Autodesk Fusion 360 part; units mm, degrees
note: some values were not read from the file. Set by a fixed rule: which sketch regions a step uses.
(part 3 of 3)
  constraint coincident P15 L924
  constraint tangent L923 A420
  constraint tangent L924 A420
  constraint tangent L926 A421
  constraint tangent L927 A421
  constraint equal A420 A421
  constraint coincident P17 L925
  constraint coincident P17 L926
  constraint tangent L925 A422
  constraint tangent L926 A422
  constraint equal A420 A422
  constraint coincident P16 L924
  constraint coincident P16 L925
  constraint tangent L924 A423
  constraint tangent L925 A423
  constraint equal A420 A423
  constraint tangent A79 L932
  constraint concentric A411 A424
  constraint tangent A413 A424
  constraint concentric A417 A427
  constraint concentric A418 A426
  constraint concentric A419 A425
  constraint concentric A412 A428
  constraint vertical L933
  constraint tangent A424 L934
  constraint vertical L934
  constraint perpendicular L929 L935
  constraint tangent L936 A426
  constraint coincident L938.start A428
  constraint tangent L938 A428
  constraint horizontal L938
  constraint concentric A428 A429
  constraint tangent L933 A430
  constraint tangent A427 A430
  constraint tangent L933 A431
  constraint tangent A426 A431
  constraint tangent L935 A432
  constraint tangent A425 A432
  constraint tangent L934 A433
  constraint tangent L935 A433
  constraint tangent L943 A441
  constraint perpendicular L926 L943
  constraint tangent L944 A441
  constraint perpendicular L926 L944
  constraint tangent L945 A443
  constraint tangent L946 A443
  constraint concentric A416 A448
  constraint tangent L937 A448
  constraint tangent A429 L951
  constraint vertical L951
  constraint perpendicular L951 L952
  constraint tangent L952 A449
  constraint tangent A448 A449
  constraint tangent L951 A450
  constraint tangent L952 A450
  constraint perpendicular L966 L967
  constraint perpendicular L963 L967
  constraint perpendicular L964 L966
  constraint tangent L966 A469
  constraint tangent A469 L967
  constraint tangent L964 A468
  constraint tangent A468 L965
  constraint equal A468 A469
  constraint tangent L963 A467
  constraint tangent A467 L964
  constraint equal A467 A469
  constraint tangent L967 A470
  constraint tangent L963 A470
  constraint equal A469 A470
  constraint tangent L974 A478
  constraint perpendicular L964 L974
  constraint tangent A478 L975
  constraint perpendicular L964 L975
  constraint tangent L972 A476
  constraint tangent A476 L973
  constraint horizontal L977
  constraint vertical L978
  constraint horizontal L979
  constraint vertical L976
  constraint concentric A483 A492
  constraint concentric A480 A491
  constraint concentric A489 A494
  constraint concentric A486 A493
  constraint tangent L976 A482
  constraint tangent A482 A483
  constraint tangent A483 A484
  constraint tangent A484 L977
  constraint equal A482 A484
  constraint tangent A481 L976
  constraint tangent A480 A481
  constraint equal A481 A482
  constraint tangent A479 L979
  constraint tangent A479 A480
  constraint equal A479 A482
  constraint tangent A490 L979
  constraint tangent A489 A490
  constraint equal A482 A490
  constraint tangent L978 A488
  constraint tangent A488 A489
  constraint equal A482 A488
  constraint tangent A486 A487
  constraint tangent A487 L978
  constraint equal A482 A487
  constraint tangent A485 A486
  constraint tangent L977 A485
  constraint equal A482 A485
  constraint horizontal L984
  constraint vertical L985
  constraint horizontal L986
  constraint vertical L987
  constraint tangent L987 A511
  constraint tangent L984 A511
  constraint tangent L986 A512
  constraint tangent L987 A512
  constraint equal A511 A512
  constraint tangent L985 A513
  constraint tangent L986 A513
  constraint equal A511 A513
  constraint tangent L984 A514
  constraint tangent L985 A514
  constraint equal A511 A514
  measures "d35" radius of A2
  measures "d36" radius of A3
  measures "d40" distance of L16.start L16.end
  measures "d41" radius of A4
  measures "d67" radius of A23
  measures "d68" distance of L75.start L75.end
  measures "d69" radius of A27
  measures "d89" radius of A39
  measures "d94" radius of A40
  measures "d112" diameter of A42
  measures "d113" diameter of A43
  measures "d116" radius of A46
  measures "d369" radius of A64
  measures "d426" diameter of A86
  measures "d427" diameter of A87
  measures "d429" radius of A88
  measures "d466" radius of A92
  measures "d474" radius of A94
  measures "d508" radius of A96
  measures "d524" diameter of A103
  measures "d525" diameter of A102
  measures "d526" radius of A104
  measures "d527" radius of A106
  measures "d528" radius of A108
  measures "d529" radius of A110
  measures "d532" distance of L341.start L341.end
  measures "d533" distance of L341.start L343.end
  measures "d534" distance of L345.start L345.end
  measures "d535" distance of L345.start L347.end
  measures "d545" radius of A116
  measures "d546" radius of A118
  measures "d555" radius of A130
  measures "d557" radius of A139
  measures "d579" radius of A171
  measures "d589" distance of L564.start L564.end
  measures "d591" radius of A172
  measures "d592" radius of A173
  measures "d593" radius of A174
  measures "d594" radius of A175
  measures "d604" radius of A182
  measures "d605" radius of A183
  measures "d643" radius of A186
  measures "d648" radius of A194
  measures "d652" radius of A205
  measures "d654" radius of A224
  measures "d655" radius of A225
  measures "d675" radius of A228
  measures "d686" radius of A230
  measures "d687" radius of A232
  measures "d688" distance of L676.start L713.end
  measures "d693" diameter of A273
  measures "d694" diameter of A274
  measures "d695" diameter of A275
  measures "d701" diameter of A276
  measures "d703" diameter of A278
  measures "d704" diameter of A279
  measures "d705" diameter of A280
  measures "d706" diameter of A281
  measures "d707" diameter of A282
  measures "d709" radius of A283
  measures "d718" diameter of A298
  measures "d719" diameter of A299
  measures "d722" radius of A300
  measures "d726" diameter of A308
  measures "d727" diameter of A309
  measures "d728" diameter of A310
  measures "d729" radius of A311
  measures "d742" radius of A348
  measures "d772" diameter of A369
  measures "d773" radius of A371
  measures "d774" radius of A381
  measures "d861" diameter of A394
  measures "d862" diameter of A395
  measures "d863" diameter of A396
  measures "d864" diameter of A397
  measures "d865" radius of A402
  measures "d872" diameter of A410
  measures "d873" diameter of A411
  measures "d876" diameter of A412
  measures "d882" radius of A413
  measures "d899" distance of L923.start P15
  measures "d901" distance of P16 P17
  measures "d902" radius of A420
  measures "d910" diameter of A427
  measures "d912" diameter of A426
  measures "d913" diameter of A425
  measures "d914" diameter of A428
  measures "d916" radius of A432
  measures "d918" radius of A433
  measures "d921" diameter of A440
  measures "d922" diameter of A441
  measures "d923" diameter of A442
  measures "d924" diameter of A443
  measures "d925" radius of A449
  measures "d926" radius of A450
  measures "d927" radius of A469
  measures "d928" diameter of A477
  measures "d929" diameter of A478
  measures "d930" diameter of A475
  measures "d931" diameter of A476
  measures "d932" diameter of A492
  measures "d933" diameter of A493
  measures "d934" diameter of A491
  measures "d935" diameter of A494
  measures "d936" radius of A482
  measures "d937" radius of A511
extrude "Estrusione12" add sketch "Schizzo1" along normal blind 5 contours L4 L5 L6 L7 A0 A1 A3 L16 L17 L18 L19 A4 A5 A6 L24 A7 L25 L26 L27 L28 A8 L29 A9 L30 A10 L31 A11 L40 A12 L41 A13 L42 A14 L43 A15 L44 L45 L54 L55 L56 L57 L58 L59 A16 L60 A17 L61 A18 L62 A19 L63 A20 L559 L560 L831 L832 L833 L834 L835 L836 | L8 L9 A2 L10 L11 L12 L13 L14 L15 L80 A31 L81 L82 L83 L84 L85 L86 L87 L88 L89 A32 L90 L91 A33 L98 L99 L100 L349 L350 L589 L590 A178 L591 A179 L595 L596 A180 L597 A181 L598 L599 L600 L601 L602 L603 | L72 L73 L75 A21 A22 A23 A24 A25 L76 L77 A26 A27 L78 L79 A28 A29 A30 L142 L143 L144 L351 L352 L353 A112 A113 A114 A115 L354 L355 L356 L357 L358 A116 A117 A118 A119 L359 A120 L360 A121 L361 A122 A123 L362 L363 A124 A125 L364 A126 A127 L365 L561 L805 A322 L806 A323 L807 A324 A325 L808 A326 A327 L809 A328 L810 A329 L811 A330 L812 A331 L813 A332 L814 A333 L815 A334 L816 L817 A335 L818 A336 L819 A337 L820 A338 L821 A339 L822 A340 L823 A341 L824 A342 A343 L825 A344 A345 L826 A346 L827 A347 L828 L829 L830 L881 L882 L883 A381 A382 L887 A387 L892 L893 A388 L894 L895 L896 A389 A390 L899 L900 L903 L905 L906 L909 L910 L913 | L101 L102 L103 L105 L106 L107 L108 L109 L110 L111 A34 L112 L113 L114 L115 L116 L117 L118 L121 A35 A36 A37 L123 L124 L125 L126 L127 L128 L129 L130 L131 A38 L133 L134 L135 L136 A39 A40 A41 L333 L334 L580 L581 L582 A176 L583 A177 L584 L587 | L307 L308 L309 L310 L311 A79 L312 L313 L314 L316 L317 L318 L319 L320 L321 L562 L563 L745 L746 L769 L770 L771 L772 L773 L774 L775 L776 L777 L778 L779 L780 L781 A295 A296 L782 L783 L784 L785 A297 L786 L787 A370 A371 A372 A373 A374 A375 A377 A378 L932 | L573 L574 L576 L577 A172 A173 A174 A175 A221 A222 A223 A224 A225 A227 A228 A229 | L640 L641 L642 L643 L644 A182 A183 A184 A185 A186 | L757 A291 L760 makes body 1 at (-47.3577, 0, -8.3435) makes body 2 at (-317.2252, 0, 47.3333) makes body 3 at (-83.3644, 0, 38.8224) makes body 4 at (33.2673, 0, -128.6547) makes body 5 at (-219.7749, 0, -101.6667) makes body 6 at (5, 0, 54.7069) makes body 7 at (26.6667, 0, 43.6243)
extrude "Extrude20" add sketch "Schizzo1" along normal blind 2 separate body contours A412 L919 L920 A413 A414 A415 A424 L933 L934 L935 L936 L937 A425 A426 A427 L938 A428 A429 A430 A431 A432 A433 L951 L952 A448 A449 A450 A451 L953 A452 A453 L954 A454 L955 A455 A456 L956 A457 A458 L957 A459 A460 L958 A461 A462 L959 A463 L960 A464 L961 A465 A466 L962 makes body 8
move_body "Move74" bodies 3 to x (1, 0, 0) y (0, 0, 1) z (0, -1, 0) at (0, 64, 54)
move_body "Move75" bodies 3 to x (1, 0, 0) y (0, 1, 0) z (0, 0, 1) at (4, 65, -64)
copy_body "CopyPasteBodies26" bodies 3 makes body 9
move_body "Move76" bodies 9 to x (1, 0, 0) y (0, 1, 0) z (0, 0, 1) at (0, 0, -135)
move_body "Move77" bodies 4 to x (0, -1, 0) y (1, 0, 0) z (0, 0, 1) at (90, 100, 0)
move_body "Move78" bodies 4 to x (1, 0, 0) y (0, 1, 0) z (0, 0, 1) at (-96, -5, 0)
move_body "Move79" bodies 2 to x (0, 0, 1) y (-1, 0, 0) z (0, -1, 0) at (-260.5, 118.5, 379)
move_body "Move80" bodies 2 to x (1, 0, 0) y (0, 1, 0) z (0, 0, 1) at (124.5, -5, -188.5)
move_body "Move81" bodies 8 to x (1, 0, 0) y (0, 0, 1) z (0, -1, 0) at (0, 77.5, 77.5)
move_body "Move82" bodies 8 to x (1, 0, 0) y (0, 1, 0) z (0, 0, 1) at (-113.75, 68.25, -82.5)
move_body "Move83" bodies 8 to x (1, 0, 0) y (0, 1, 0) z (0, 0, 1) at (-1, 0, 0)
copy_body "CopyPasteBodies27" bodies 8 makes body 10
move_body "Move84" bodies 10 to x (1, 0, 0) y (0, 1, 0) z (0, 0, 1) at (0, 0, -142)
move_body "Move86" bodies 8 to x (0, 0, -1) y (0, 1, 0) z (1, 0, 0) at (-81.75, 0, -87.75)
move_body "Move87" bodies 8 to x (1, 0, 0) y (0, 1, 0) z (0, 0, 1) at (-49.25, -2.75, -61)
move_body "Move88" bodies 8 to x (1, 0, 0) y (0, 1, 0) z (0, 0, 1) at (0, 3, 3)
move_body "Move89" bodies 5 to x (1, 0, 0) y (0, 1, 0) z (0, 0, 1) at (196, 70, 0)
copy_body "CopyPasteBodies29" bodies 10 makes body 11
move_body "Move90" bodies 11 to x (1, 0, 0) y (0, 1, 0) z (0, 0, 1) at (0, 0, 142)
